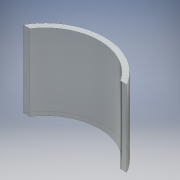
# Autodesk Inventor part: outsideCover2
Saved by Autodesk Inventor 2016 (Build 200138000, 138)
## iProperties
Created: 2016-11-11
Part Number: outsideCover2
Material: ガラス
Document SubType Name: Modeling
Designer: Daisuke
Density: 2.18 g/cm^3
Appearance: クリア
Author: Daisuke
Autodesk Inventor part; units mm, degrees
ref_plane "YZ Plane" through (0, 0, 0) normal (1, 0, 0) x (0, 1, 0)
ref_plane "XZ Plane" through (0, 0, 0) normal (0, 1, 0) x (-1, 0, 0)
ref_plane "XY Plane" through (0, 0, 0) normal (0, 0, 1) x (1, 0, 0)
sketch "スケッチ1" plane through (0, 0, 0) normal (0, 0, 1) x (1, 0, 0)
  line L0 (0, 0) -> (47.6314, 27.5) construction
  line L1 (50, 0) -> (55, 0) construction
  line L2 (0, 0) -> (-47.6314, 27.5) construction
  line L3 (0, 0) -> (55, 0) construction
  line L4 (-47.6314, 27.5) -> (-41.7582, 27.5)
  line L5 (41.7582, 27.5) -> (47.6314, 27.5)
  line L6 (0, 0) -> (55, 0) construction
  line L7 (0, 0) -> (55, 0) construction
  arc A0 (47.6314, 27.5) -> (-47.6314, 27.5) centre (0, 0) ccw
  arc A1 (41.7582, 27.5) -> (-41.7582, 27.5) centre (0, 0) ccw
  arc A2 (47.6314, 27.5) -> (-47.6314, 27.5) centre (0, 0) ccw construction
  dimension "d0" = 30
  dimension "d1" = 150
  constraints: 16 end point, 6 point on circle, 4 horizontal, 3 centre point, 2 coincident, 1 equal length
  measures "d0" angle of L1 L0
  measures "d1" angle of L3 L2
extrude "押し出し1" add sketch "スケッチ1" along normal blind 70.5
